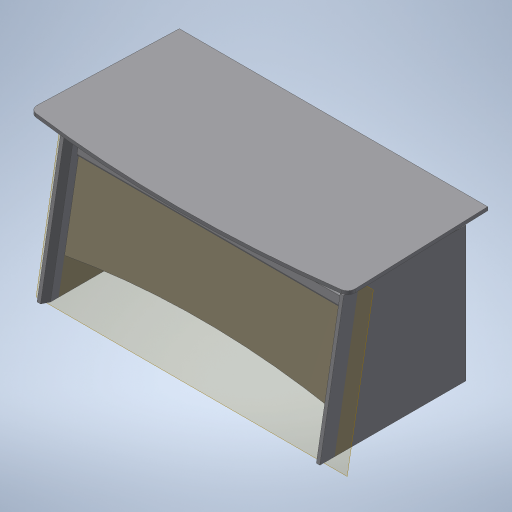
# Autodesk Inventor part: Table
Saved by Autodesk Inventor 2024 (Build 280153000, 153)
## iProperties
Created: 2013-10-09
Part Number: Table
Material: Generic
Document SubType Name: Modeling
Designer: SauliusD
Density: 1 g/cm^3
Appearance: Default
Author: SauliusD
Autodesk Inventor part; units mm, degrees
ref_plane "YZ Plane" through (0, 0, 0) normal (1, 0, 0) x (0, 1, 0)
ref_plane "XZ Plane" through (0, 0, 0) normal (0, 1, 0) x (-1, 0, 0)
ref_plane "XY Plane" through (0, 0, 0) normal (0, 0, 1) x (1, 0, 0)
sketch "Sketch1" plane through (0, 0, 0) normal (0, 0, 1) x (1, 0, 0)
  line L0 (-775, -400) -> (775, -400)
  line L1 (775, -400) -> (775, 400)
  line L2 (775, 400) -> (-775, 400)
  line L3 (-775, 400) -> (-775, -400)
  line L4 (-775, -400) -> (775, 400) construction
  line L5 (775, -400) -> (-775, 400) construction
  point P0 (0, 0)
  dimension "d0" = 1550
  dimension "d1" = 800
  constraints: 12 end point, 2 midpoint, 2 parallel, 1 horizontal, 1 perpendicular
  measures "d0" distance of L2.end L1.end
  measures "d1" distance of L1.end L0.end
extrude "Extrusion1" add sketch "Sketch1" along normal blind 800
draft "FaceDraft1" angle -10 pull direction (0, 0, -1) faces at (-258.333333, -400, 266.666667) fixed edges at (0, -400, 0)
sketch "Sketch2" plane through (0, 0, 800) normal (0, 0, 1) x (1, 0, 0)
  line L0 (775, 400) -> (-775, 400)
  line L1 (-775, 400) -> (-775, -258.938415)
  line L2 (-875, 450) -> (875, 450)
  line L3 (875, 450) -> (875, -400)
  line L4 (875, -400) -> (-875, -400)
  line L5 (-875, -400) -> (-875, 450)
  line L6 (-775, -400) -> (775, -400)
  point P0 (0, 0)
  point P1 (0, 450)
  dimension "d5" = 50
  dimension "d6" = 100
  constraints: 8 end point, 2 parallel, 1 collinear, 1 horizontal, 1 midpoint, 1 perpendicular, 1 vertical alignment
  measures "d5" distance between parallel lines of L0 L2
  measures "d6" distance between parallel lines of L5 L1
extrude "Extrusion2" add sketch "Sketch2" along normal blind 37 separate body
sketch "Sketch3" plane through (0, 0, 837) normal (0, 0, 1) x (1, 0, 0)
  line L0 (875, 450) -> (-875, 450) projected
  line L1 (875, -400) -> (875, 450) projected
  line L2 (845, 450) -> (875, -400)
  point P0 (0, 0)
  dimension "d10" = 30
  constraints: 2 end point, 1 point on line
  measures "d10" distance from line of L1 L2.start
extrude "Extrusion3" cut sketch "Sketch3" against normal through all bodies 2
mirror "Mirror1" about plane through (0, 0, 0) normal (1, 0, 0) of "Extrusion3" bodies 2
sketch "Sketch4" plane through (0, 0, 837) normal (0, 0, 1) x (1, 0, 0)
  line L0 (-845, 450) -> (-875, -400)
  line L1 (-875, -400) -> (875, -400)
  line L2 (875, -400) -> (845, 450)
  line L3 (845, 450) -> (-845, 450)
  arc A0 (-872.882353, -340) -> (872.882353, -340) centre (0, 5979.363351) ccw
  point P0 (0, 0)
  dimension "d13" = 60
  constraints: 2 point on circle, 2 point on line, 1 centre point, 1 horizontal alignment, 1 tangent
  measures "d13" distance from line of L1 A0.start
extrude "Extrusion4" cut sketch "Sketch4" against normal through all contours A0 L1 L0 | A0 L2 L1 bodies 2
move faces "Move Face1" translate (0, 0, -60) faces at (258.333333, -39.292277, 800)
sketch "Sketch5" plane through (-775, -400, 0) normal (-1, 0, 0) x (0, 0, 1)
  line L0 (0, 800) -> (0, 0)
  line L1 (0, 0) -> (740, 130.481966)
  line L2 (740, 800) -> (740, 130.481966)
  line L3 (0, 800) -> (740, 800)
  point P0 (0, 400)
extrude "Extrusion5" add sketch "Sketch5" against normal blind 37 separate body
mirror "Mirror2" about plane through (0, 0, 0) normal (1, 0, 0) bodies 3 separate body
ref_plane "Work Plane1" through (-775, -321.21538, -13.891854) normal (0, -0.9848078, 0.1736482) x (1, 0, 0)
sketch "Sketch6" plane through (-775, -321.21538, -13.891854) normal (0, -0.9848078, 0.1736482) x (1, 0, 0)
  line L0 (37, 138.918542) -> (37, 867.676279) construction
  line L1 (1513, 138.918542) -> (1513, 867.676279) construction
  line L2 (37, 691.415693) -> (1513, 691.415693)
  line L3 (1513, 691.415693) -> (1513, 200)
  line L4 (1513, 200) -> (37, 200)
  line L5 (37, 200) -> (37, 691.415693)
  line L6 (0, 751.415693) -> (1550, 751.415693)
  line L7 (0, 0) -> (1550, 0)
  arc A0 (1513, 200) -> (37, 200) centre (775, -4308.7) ccw
  line L8 (381.15741, 260) -> (1087.694137, 260) construction
  point P0 (775, 69.459271)
  dimension "d20" = 60
  dimension "d21" = 200
  dimension "d22" = 60
  constraints: 10 end point, 3 parallel, 2 point on circle, 2 point on line, 1 centre point, 1 horizontal, 1 perpendicular, 1 tangent
  measures "d20" distance between parallel lines of L2 L6
  measures "d21" distance between parallel lines of L7 L4
  measures "d22" distance between parallel lines of L4 L8
extrude "Extrusion6" add sketch "Sketch6" against normal blind 18 separate body contours L2 L3 A0 L5
sketch "Sketch7" plane through (-738, -400, 0) normal (1, 0, 0) x (0, 0, -1)
  line L0 (0, 800) -> (-740, 800) construction
  line L1 (-179.944029, 131.240795) -> (-663.894013, 216.574235) construction
  line L2 (-800, 60) -> (-800, 60) construction
  line L3 (-800, 60) -> (-800, 850) construction
  line L4 (-800, 850) -> (-800, 60) construction
  line L5 (-279.944029, 148.873493) -> (-800, 240.573393)
  line L6 (-800, 240.573393) -> (-800, 740)
  line L7 (-800, 740) -> (-279.944029, 740)
  line L8 (-279.944029, 740) -> (-279.944029, 148.873493)
  point P0 (0, 400)
  dimension "d25" = 60
  dimension "d26" = 100
  constraints: 8 end point, 3 point on line, 2 perpendicular, 1 collinear, 1 parallel
  measures "d25" distance between parallel lines of L0 L7
  measures "d26" distance from line of L1.start L8
extrude "Extrusion7" add sketch "Sketch7" along normal blind 18 separate body
mirror "Mirror3" about plane through (0, 0, 0) normal (1, 0, 0) bodies 6 separate body
fillet "Fillet1" radius 40 2 edges at (-872.8824, -340, 818.5) (872.8824, -340, 818.5)
sketch "Sketch8" plane through (738, -201.152305, 667.019681) normal (1, 0, 0) x (0, -0.1736482, -0.9848078)
  line L0 (491.415693, 0) -> (0, 0)
  line L1 (0, 18) -> (-10, 18)
  line L2 (-10, 18) -> (-10, -10)
  line L3 (-10, -10) -> (0, -10)
  line L4 (0, -10) -> (0, 18)
  line L5 (0, -10) -> (50, -10)
  line L6 (50, -10) -> (50, 0)
  line L7 (50, 0) -> (0, 0)
  line L8 (0, 0) -> (0, -10)
  point P0 (621.956422, 313.923101)
  dimension "d30" = 60
  dimension "d31" = 10
  constraints: 16 end point, 4 parallel, 3 perpendicular, 2 horizontal, 1 point on line
  measures "d30" distance between parallel lines of L6 L2
  measures "d31" distance of L1.start L1.end
extrude "Extrusion8" add sketch "Sketch8" against normal up to surface (1476 mm away) separate body
fillet "Fillet2" radius 10 2 edges at (0, -209.2639, 678.6042) (0, -219.6828, 619.5158)
chamfer "Chamfer1" distance 36 distance2 18 5 edges at (858.3024, 73.0982, 800) (862.1724, -331.0437, 800) (0, -400, 800) (-862.1724, -331.0437, 800) (-858.3024, 73.0982, 800) measured on face at (0, -399.5, 800) measured on face at (857.8027, 73.0805, 800) measured on face at (-861.7906, -330.7208, 800) measured on face at (-857.8027, 73.0805, 800) measured on face at (861.7906, -330.7208, 800)
chamfer "Chamfer2" distance 36 distance2 18 1 edges at (-738, -334.759, 370) measured on face at (-738, -334.2666, 369.9132)
chamfer "Chamfer3" distance 18 distance2 36 1 edges at (738, -334.759, 370) measured on face at (738.5, -334.759, 370)
body "Solid1"
